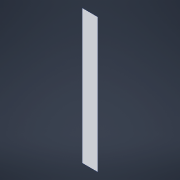
# Autodesk Inventor part: StarBackdropPanel
Saved by Autodesk Inventor 2021 (Build 250183000, 183)
## iProperties
Created: 2021-01-31
Part Number: StarBackdropPanel
Material: Generic
Document SubType Name: Modeling
Designer: argon
Density: 1 g/cm^3
Appearance: Ice White
Author: argon
Autodesk Inventor part; units mm, degrees
ref_plane "YZ Plane" through (0, 0, 0) normal (1, 0, 0) x (0, 1, 0)
ref_plane "XZ Plane" through (0, 0, 0) normal (0, 1, 0) x (-1, 0, 0)
ref_plane "XY Plane" through (0, 0, 0) normal (0, 0, 1) x (1, 0, 0)
sketch "Sketch1" plane through (0, 0, 0) normal (0, 0, 1) x (1, 0, 0)
  line L0 (-695.173, 6000) -> (695.173, 6000)
  line L1 (695.173, 6000) -> (695.173, -6000)
  line L2 (695.173, -6000) -> (-695.173, -6000)
  line L3 (-695.173, -6000) -> (-695.173, 6000)
  line L4 (-695.173, 6000) -> (695.173, -6000) construction
  line L5 (695.173, 6000) -> (-695.173, -6000) construction
  point P0 (0, 0)
  dimension "d0" = 1390.346
  dimension "d1" = 12000
  constraints: 12 end point, 2 midpoint, 2 parallel, 1 horizontal, 1 perpendicular
  measures "d0" distance of L1.end L2.end
  measures "d1" distance of L0.end L1.end
extrude "Extrusion1" add sketch "Sketch1" along normal blind 9
body "Solid1"
